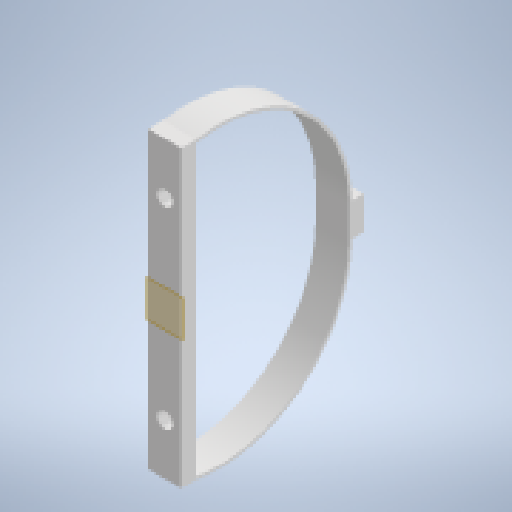
# Autodesk Inventor part: MotorMountBackSuspension
Saved by Autodesk Inventor 2024 (Build 280153020, 153B)
## iProperties
Created: 2024-04-18
Part Number: MotorMountBackSuspension
Material: Generic
Document SubType Name: Modeling
Designer: lvrectanus0
Density: 1 g/cm^3
Appearance: Default
Author: lvrectanus0
Autodesk Inventor part; units mm, degrees
ref_plane "YZ Plane" through (0, 0, 0) normal (1, 0, 0) x (0, 1, 0)
ref_plane "XZ Plane" through (0, 0, 0) normal (0, 1, 0) x (-1, 0, 0)
ref_plane "XY Plane" through (0, 0, 0) normal (0, 0, 1) x (1, 0, 0)
sketch "Sketch1" plane through (0, 0, 0) normal (0, 0, 1) x (1, 0, 0)
  circle A0 centre (0, 0) radius 2 projected
  arc A1 (3.5334, 2.622) -> (3.5334, -2.622) centre (0, 0) ccw projected
  spline S0 degree 3 poles (3.5334, -2.622) (3.7278, -2.3601) (3.9365, -2.0888) (4.2711, -1.5149) (4.4221, -1.1997) (4.5595, -0.6718) (4.5884, -0.5166) (4.6147, -0.2815) (4.6206, -0.2033) (4.626, -0.0622) (4.6266, 0.0005) (4.624, 0.1338) (4.6203, 0.2042) (4.6043, 0.3928) (4.5877, 0.5103) (4.479, 1.0643) (4.3163, 1.4256) (3.965, 2.0517) (3.7411, 2.3422) (3.5334, 2.622) knots 0 0 0 0 0.091406 0.091406 0.164876 0.164876 0.194861 0.194861 0.209742 0.209742 0.221646 0.221646 0.235028 0.235028 0.25755 0.25755 0.34212 0.34212 0.446672 0.446672 0.446672 0.446672 projected
  line L0 (4.4, -4.4) -> (-4.4, -4.4)
  line L1 (-4.4, -4.4) -> (-4.4, 4.4)
  line L2 (-4.4, 4.4) -> (4.4, 4.4)
  line L3 (4.4, 4.4) -> (4.4, -4.4)
  line L4 (4.4, -4.4) -> (-4.4, 4.4) construction
  line L5 (-4.4, -4.4) -> (4.4, 4.4) construction
  point P0 (0, 0)
  constraints: 12 end point, 2 midpoint, 2 parallel, 2 tangent, 1 horizontal, 1 perpendicular
extrude "Extrusion1" add sketch "Sketch1" along normal blind 4 contours A0 | S0 L3 A1 | A1 L2 L3 S0 | A1 L1 L2 | A1 L0 L1 | L3 L0 A1 S0
ref_plane "Work Plane1" through (-30.8084, 0, 48.1765) normal (0, 0, 1) x (1, 0, 0)
sketch "Sketch2" plane through (-30.8084, 0, 48.1765) normal (0, 0, 1) x (1, 0, 0)
  line L0 (35.2084, 38.1) -> (26.4084, 38.1)
  line L1 (26.4084, 38.1) -> (26.4084, -38.1)
  line L2 (26.4084, -38.1) -> (35.2084, -38.1)
  line L3 (35.2084, -38.1) -> (35.2084, 38.1)
  line L4 (35.2084, 38.1) -> (26.4084, -38.1) construction
  line L5 (26.4084, 38.1) -> (35.2084, -38.1) construction
  line L6 (35.2084, 4.4) -> (26.4084, 4.4) projected
  line L7 (26.4084, 4.4) -> (26.4084, -4.4) projected
  line L8 (26.4084, -4.4) -> (35.2084, -4.4) projected
  line L9 (35.2084, -4.4) -> (35.2084, 4.4) projected
  line L10 (35.2084, -38.1) -> (26.4084, -38.1)
  line L11 (26.4084, -38.1) -> (26.4084, -38.9)
  line L12 (26.4084, -38.9) -> (35.2084, -38.9)
  line L13 (35.2084, -38.9) -> (35.2084, -38.1)
  line L14 (35.2084, 38.1) -> (26.4084, 38.1)
  line L15 (26.4084, 38.1) -> (26.4084, 38.9)
  line L16 (26.4084, 38.9) -> (35.2084, 38.9)
  line L17 (35.2084, 38.9) -> (35.2084, 38.1)
  point P0 (30.8084, 0)
  point P1 (26.4084, 0)
  point P2 (26.4084, -38.1)
  dimension "d2" = 38.1
  dimension "d8" = 0.8
  dimension "d9" = 0.8
  constraints: 28 end point, 6 parallel, 4 midpoint, 3 horizontal, 3 perpendicular, 1 point on line, 1 vertical alignment
  measures "d2" distance from line of L2 point (30.808, 0)
  measures "d8" distance of L11.end L10.end
  measures "d9" distance of L14.end L15.end
sketch "Sketch4" plane through (-4.4, 4.4, 0) normal (0, 1, 0) x (1, 0, 0)
  line L0 (8.8, 0) -> (8.8, -4) projected
  line L1 (0, 0) -> (0, -4) projected
  line L2 (8.8, -4) -> (0, -4)
  line L3 (0, -4) -> (0, -3.2)
  line L4 (0, -3.2) -> (8.8, -3.2)
  line L5 (8.8, -3.2) -> (8.8, -4)
  point P0 (4.4, 0)
  dimension "d3" = 0.8
  constraints: 8 end point, 2 parallel, 1 horizontal, 1 perpendicular, 1 point on line
  measures "d3" distance of L2.end L3.end
extrude "Extrusion2" add sketch "Sketch2" against normal blind 4
sketch "Sketch3" plane through (4.4, -4.4, 0) normal (1, 0, 0) x (0, 0, -1)
  line L0 (-48.1765, -33.7) -> (-48.1765, 42.5) construction
  line L1 (0, 0) -> (0, 8.8) projected
  line L2 (0, 8.8) -> (-4, 8.8) projected
  line L3 (-4, 0) -> (-4, 8.8) projected
  line L4 (0, 0) -> (-4, 0) projected
  arc A0 (-44.1765, -33.7) -> (-4, 0) centre (-38.222, 0) ccw
  line L5 (-44.1765, 43.3) -> (-44.1765, -34.5) projected
  arc A1 (-4, 8.8) -> (-44.1765, 42.5) centre (-38.222, 8.8) ccw
  line L6 (-44.1765, -33.7) -> (-44.1765, 42.5)
  point P0 (0, 4.4)
  constraints: 4 point on circle, 2 centre point, 2 end point, 2 horizontal alignment, 2 tangent, 1 collinear, 1 point on line, 1 vertical alignment
sweep "Sweep2" add profiles "Sketch4" path "Sketch3" path curves A1 L6 A0
sketch "Sketch5" plane through (-30.8084, 0, 48.1765) normal (0, 0, 1) x (1, 0, 0)
  line L0 (35.2084, -38.9) -> (35.2084, 38.9) projected
  line L1 (35.2084, 38.9) -> (26.4084, 38.9) projected
  line L2 (26.4084, 38.9) -> (26.4084, -38.9) projected
  line L3 (26.4084, -38.9) -> (35.2084, -38.9) projected
  circle A0 centre (30.8084, -25.4) radius 2
  line L4 (35.2084, 0) -> (26.4084, 0)
  circle A1 centre (30.8084, 25.4) radius 2
  point P0 (30.8084, 0)
  dimension "d12" = 4
  dimension "d13" = 25.4
  constraints: 2 centre point, 2 end point, 2 midpoint, 1 symmetric about line, 1 vertical alignment, 1 other
  measures "d12" diameter of A0
  measures "d13" distance of point (30.808, 0) A0.centre
hole "Hole1" at (0, -25.4, 48.1765) at (0, 25.4, 48.1765) direction (0, 0, -1) diameter 4 depth 6
body "Solid1"
